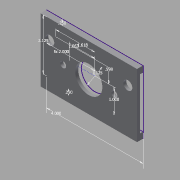
# Autodesk Inventor part: Mounting Jig
Saved by Autodesk Inventor 2013 (Build 170138000, 138)
## iProperties
Created: 2013-10-22
Part Number: Mounting Jig
Material: Generic
Document SubType Name: Modeling
Designer: grtstudent
Density: 1 g/cm^3
Author: grtstudent
Autodesk Inventor part; units mm, degrees
ref_plane "YZ Plane" through (0, 0, 0) normal (1, 0, 0) x (0, 1, 0)
ref_plane "XZ Plane" through (0, 0, 0) normal (0, 1, 0) x (-1, 0, 0)
ref_plane "XY Plane" through (0, 0, 0) normal (0, 0, 1) x (1, 0, 0)
sketch "Sketch1" plane through (0, 0, 0) normal (0, 0, 1) x (1, 0, 0)
  line L0 (0, 0) -> (101.6, 0)
  line L1 (101.6, 0) -> (101.6, 53.975)
  line L2 (101.6, 53.975) -> (0, 53.975)
  line L3 (0, 53.975) -> (0, 0)
  circle A0 centre (50.8, 25.4) radius 14.2875
  line L4 (23.8125, 25.4) -> (50.8, 25.4) construction
  line L5 (50.8, 25.4) -> (77.7875, 25.4) construction
  line L6 (50.8, 25.4) -> (50.8, 53.975) construction
  line L7 (101.6, 0) -> (101.6, -6.35)
  line L8 (101.6, -6.35) -> (0, -6.35)
  line L9 (0, -6.35) -> (0, 0)
  line L10 (0, 53.975) -> (101.6, 53.975)
  line L11 (101.6, 53.975) -> (101.6, 60.325)
  line L12 (101.6, 60.325) -> (0, 60.325)
  line L13 (0, 60.325) -> (0, 53.975)
  point P0 (9.704, 40.5945)
  point P1 (91.896, 40.5945)
  dimension "d0" = 53.975
  dimension "d2" = 101.6
  dimension "d3" = 28.575
  dimension "d4" = 50.8
  dimension "d5" = 25.4
  dimension "d6" = 26.9875
  dimension "d7" = 41.096
  dimension "d8" = 15.1945
  dimension "d9" = 6.35
  dimension "d10" = 6.35
  constraints: 28 end point, 5 parallel, 4 horizontal, 3 perpendicular, 1 centre point, 1 coincident, 1 collinear, 1 midpoint, 1 symmetric about line
  measures "d0" distance of L2.end L0.start
  measures "d2" distance of L0.start L0.end
  measures "d3" diameter of A0
  measures "d4" distance from line of L3 L4.end
  measures "d5" distance from line of L0 L4.end
  measures "d6" distance of L4.end L4.start
  measures "d7" distance from line of L6 point (9.704, 40.595)
  measures "d8" vertical distance of L4.end point (9.704, 40.595)
  measures "d9" distance between parallel lines of L2 L12
  measures "d10" distance between parallel lines of L0 L8
extrude "Extrusion1" add sketch "Sketch1" along normal blind 6.35
extrude "Extrusion2" cut sketch "Sketch1" along normal blind 3.175 contours L3 L2 L1 L0
hole "Hole1" at (23.8125, 25.4, 0) at (77.7875, 25.4, 0) direction (0, 0, 1) diameter 6.35 end through all
hole "Hole2" at (9.704, 40.5945, 0) at (91.896, 40.5945, 0) direction (0, 0, 1) diameter 9.525 end through all
equation "\"d4\" = 0.5 * d2"
body "Solid1"
